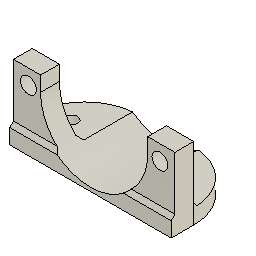
Motor Clip (Autodesk Fusion 360 design; units mm, degrees)
Autodesk Fusion 360 part; units mm, degrees
sketch "Sketch1" plane through (0, 0, 0) normal (0, 1, 0) x (1, 0, 0)
  line L0 (-21.4929, -3.9767) -> (-14.25, -3.9767)
  arc A0 (14.25, 0) -> (-14.25, 0) centre (0, 0) ccw
  line L1 (-21.4929, -3.9767) -> (-21.4929, 15.251)
  line L2 (21.5026, 15.251) -> (-21.4929, 15.251)
  circle A1 centre (-17.5048, 0.0114) radius 2.1
  line L3 (21.5026, -4.0254) -> (14.25, -4.0217)
  circle A2 centre (17.4952, -0.0012) radius 2.1
  line L4 (21.5026, -4.0254) -> (21.5026, 15.251)
  line L5 (-21.4929, 11.251) -> (-8.7451, 11.251)
  line L6 (8.7451, 11.251) -> (21.5026, 11.251)
  line L7 (-14.25, -3.9767) -> (-14.25, 0)
  line L8 (14.25, 0) -> (14.25, -4.0217)
  dimension "d1" = 28.5
  dimension "d4" = 4.2
  dimension "d14" = 4
  dimension "d33" = 35
  dimension "d34" = 4.2
  measures "d1" diameter of A0
  measures "d4" diameter of A1
  measures "d14" distance of L2 L5
  measures "d34" diameter of A2
extrude "Extrude1" add sketch "Sketch1" along normal blind 5 from surface at 1
extrude "Extrude3" add sketch "Sketch1" along normal blind 20 contours A0 L1 L2 L4 L5 L6
sketch "Sketch4" plane through (0, 0, -15.251) normal (0, 0, -1) x (1, 0, 0)
  line L0 (-21.4929, 0) -> (-21.4929, -20)
  line L1 (-21.4929, -20) -> (21.5026, -20)
  line L2 (21.5026, -20) -> (21.5026, 0)
  line L3 (-21.4929, 0) -> (-21.4929, -20)
  line L4 (-21.4929, -20) -> (21.5026, -20)
  line L5 (21.5026, -20) -> (21.5026, 0)
  line L6 (21.5026, 0) -> (-21.4929, 0)
  circle A0 centre (-14.9976, -10) radius 1.6
  line L7 (0.0024, 3.9978) -> (0.0024, -22.1306)
  circle A1 centre (15.0024, -10) radius 1.6
  dimension "d50" = 3.2
  dimension "d51" = 10
  dimension "d52" = 15
  measures "d50" diameter of A0
  measures "d52" distance of L7
extrude "Extrude8" cut sketch "Sketch4" along normal blind -8 and the other way blind -2 contours A0 | A1
chamfer "Chamfer1" distance 1 angle 45 4 edges at (-15.119, 1, -11.251) (15.1239, 1, -11.251) (-15.119, 6, -11.251) (15.1239, 6, -11.251)
fillet "Fillet1" radius 14 2 edges at (-21.4929, 20, -13.251) (21.5026, 20, -13.251)
equation "d34 = d4"
named bodies: "Motor Clip"
